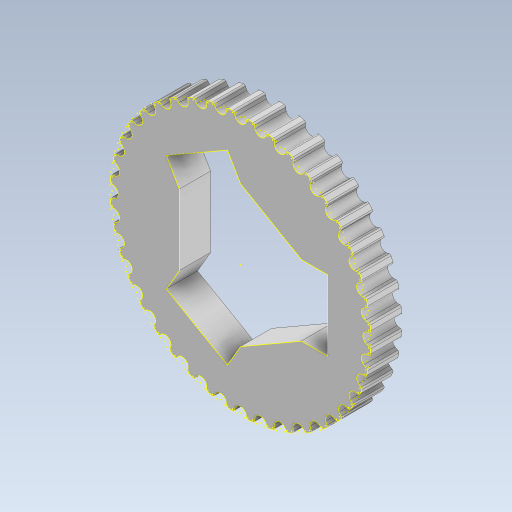
# Autodesk Inventor part: 2GT_40T
Saved by Autodesk Inventor 2023 (Build 270158000, 158)
## iProperties
Created: 2023-05-04
Part Number: 2GT_40T
Material: 一般
Document SubType Name: Modeling
Designer: Johnny Jou
Density: 1 g/cm^3
Appearance: 預設
Author: Johnny Jou
Autodesk Inventor part; units mm, degrees
ref_plane "YZ Plane" through (0, 0, 0) normal (1, 0, 0) x (0, 1, 0)
ref_plane "XZ Plane" through (0, 0, 0) normal (0, 1, 0) x (-1, 0, 0)
ref_plane "XY Plane" through (0, 0, 0) normal (0, 0, 1) x (1, 0, 0)
sketch "草圖1" plane through (0, 0, 0) normal (0, 0, 1) x (1, 0, 0)
  arc A0 (1.3466, 12.2657) -> (1.2112, 12.4161) centre (1.1966, 12.2668) ccw
  arc A1 (1.2112, 12.4161) -> (0.746, 12.4527) centre (0, 0) ccw
  arc A2 (0.746, 12.4527) -> (0.5887, 12.3254) centre (0.7371, 12.3029) ccw
  arc A3 (0.4989, 12.0368) -> (0.5887, 12.3254) centre (-0.4, 12.475) ccw
  arc A4 (-0.4989, 12.0368) -> (0.4989, 12.0368) centre (0, 12.28) ccw
  arc A5 (-0.5887, 12.3254) -> (-0.4989, 12.0368) centre (0.4, 12.475) ccw
  arc A6 (-0.5887, 12.3254) -> (-0.746, 12.4527) centre (-0.7371, 12.3029) ccw
  arc A7 (-0.746, 12.4527) -> (-1.2112, 12.4161) centre (0, 0) ccw
  arc A8 (-1.2112, 12.4161) -> (-1.3466, 12.2657) centre (-1.1966, 12.2668) ccw
  arc A9 (-1.3902, 11.9666) -> (-1.3466, 12.2657) centre (-2.3466, 12.2588) ccw
  arc A10 (-2.3757, 11.8106) -> (-1.3902, 11.9666) centre (-1.921, 12.1288) ccw
  arc A11 (-2.5096, 12.0815) -> (-2.3757, 11.8106) centre (-1.5564, 12.384) ccw
  arc A12 (-2.5096, 12.0815) -> (-2.6849, 12.1827) centre (-2.6526, 12.0362) ccw
  arc A13 (-2.6849, 12.1827) -> (-3.1386, 12.0737) centre (0, 0) ccw
  arc A14 (-3.1386, 12.0737) -> (-3.2488, 11.9041) centre (-3.1008, 11.9286) ccw
  arc A15 (-3.2451, 11.6018) -> (-3.2488, 11.9041) centre (-4.2354, 11.7408) ccw
  arc A16 (-4.194, 11.2935) -> (-3.2451, 11.6018) centre (-3.7947, 11.679) ccw
  arc A17 (-4.3687, 11.5402) -> (-4.194, 11.2935) centre (-3.4746, 11.988) ccw
  arc A18 (-4.3687, 11.5402) -> (-4.5576, 11.6127) centre (-4.5028, 11.473) ccw
  arc A19 (-4.5576, 11.6127) -> (-4.9887, 11.4341) centre (0, 0) ccw
  arc A20 (-4.9887, 11.4341) -> (-5.071, 11.2493) centre (-4.9287, 11.2966) ccw
  arc A21 (-5.0201, 10.9514) -> (-5.071, 11.2493) centre (-6.0199, 10.9337) ccw
  arc A22 (-5.9091, 10.4984) -> (-5.0201, 10.9514) centre (-5.575, 10.9416) ccw
  arc A23 (-6.1202, 10.7147) -> (-5.9091, 10.4984) centre (-5.3071, 11.2969) ccw
  arc A24 (-6.1202, 10.7147) -> (-6.3181, 10.7567) centre (-6.2421, 10.6274) ccw
  arc A25 (-6.3181, 10.7567) -> (-6.7159, 10.5129) centre (0, 0) ccw
  arc A26 (-6.7159, 10.5129) -> (-6.7684, 10.3175) centre (-6.6352, 10.3865) ccw
  arc A27 (-6.6715, 10.0312) -> (-6.7684, 10.3175) centre (-7.6562, 9.8574) ccw
  arc A28 (-7.4787, 9.4447) -> (-6.6715, 10.0312) centre (-7.218, 9.9347) ccw
  arc A29 (-7.721, 9.6254) -> (-7.4787, 9.4447) centre (-7.009, 10.3276) ccw
  arc A30 (-7.721, 9.6254) -> (-7.923, 9.6359) centre (-7.8278, 9.5201) ccw
  arc A31 (-7.923, 9.6359) -> (-8.2778, 9.3329) centre (0, 0) ccw
  arc A32 (-8.2778, 9.3329) -> (-8.2991, 9.1317) centre (-8.1783, 9.2207) ccw
  arc A33 (-8.1585, 8.8641) -> (-8.2991, 9.1317) centre (-9.104, 8.5383) ccw
  arc A34 (-8.8641, 8.1585) -> (-8.1585, 8.8641) centre (-8.6833, 8.6833) ccw
  arc A35 (-9.1317, 8.2991) -> (-8.8641, 8.1585) centre (-8.5383, 9.104) ccw
  arc A36 (-9.1317, 8.2991) -> (-9.3329, 8.2778) centre (-9.2207, 8.1783) ccw
  arc A37 (-9.3329, 8.2778) -> (-9.6359, 7.923) centre (0, 0) ccw
  arc A38 (-9.6359, 7.923) -> (-9.6254, 7.721) centre (-9.5201, 7.8278) ccw
  arc A39 (-9.4447, 7.4787) -> (-9.6254, 7.721) centre (-10.3276, 7.009) ccw
  arc A40 (-10.0312, 6.6715) -> (-9.4447, 7.4787) centre (-9.9347, 7.218) ccw
  arc A41 (-10.3175, 6.7684) -> (-10.0312, 6.6715) centre (-9.8574, 7.6562) ccw
  arc A42 (-10.3175, 6.7684) -> (-10.5129, 6.7159) centre (-10.3865, 6.6352) ccw
  arc A43 (-10.5129, 6.7159) -> (-10.7567, 6.3181) centre (0, 0) ccw
  arc A44 (-10.7567, 6.3181) -> (-10.7147, 6.1202) centre (-10.6274, 6.2421) ccw
  arc A45 (-10.4984, 5.9091) -> (-10.7147, 6.1202) centre (-11.2969, 5.3071) ccw
  arc A46 (-10.9514, 5.0201) -> (-10.4984, 5.9091) centre (-10.9416, 5.575) ccw
  arc A47 (-11.2493, 5.071) -> (-10.9514, 5.0201) centre (-10.9337, 6.0199) ccw
  arc A48 (-11.2493, 5.071) -> (-11.4341, 4.9887) centre (-11.2966, 4.9287) ccw
  arc A49 (-11.4341, 4.9887) -> (-11.6127, 4.5576) centre (0, 0) ccw
  arc A50 (-11.6127, 4.5576) -> (-11.5402, 4.3687) centre (-11.473, 4.5028) ccw
  arc A51 (-11.2935, 4.194) -> (-11.5402, 4.3687) centre (-11.988, 3.4746) ccw
  arc A52 (-11.6018, 3.2451) -> (-11.2935, 4.194) centre (-11.679, 3.7947) ccw
  arc A53 (-11.9041, 3.2488) -> (-11.6018, 3.2451) centre (-11.7408, 4.2354) ccw
  arc A54 (-11.9041, 3.2488) -> (-12.0737, 3.1386) centre (-11.9286, 3.1008) ccw
  arc A55 (-12.0737, 3.1386) -> (-12.1827, 2.6849) centre (0, 0) ccw
  arc A56 (-12.1827, 2.6849) -> (-12.0815, 2.5096) centre (-12.0362, 2.6526) ccw
  arc A57 (-11.8106, 2.3757) -> (-12.0815, 2.5096) centre (-12.384, 1.5564) ccw
  arc A58 (-11.9666, 1.3902) -> (-11.8106, 2.3757) centre (-12.1288, 1.921) ccw
  arc A59 (-12.2657, 1.3466) -> (-11.9666, 1.3902) centre (-12.2588, 2.3466) ccw
  arc A60 (-12.2657, 1.3466) -> (-12.4161, 1.2112) centre (-12.2668, 1.1966) ccw
  arc A61 (-12.4161, 1.2112) -> (-12.4527, 0.746) centre (0, 0) ccw
  arc A62 (-12.4527, 0.746) -> (-12.3254, 0.5887) centre (-12.3029, 0.7371) ccw
  arc A63 (-12.0368, 0.4989) -> (-12.3254, 0.5887) centre (-12.475, -0.4) ccw
  arc A64 (-12.0368, -0.4989) -> (-12.0368, 0.4989) centre (-12.28, 0) ccw
  arc A65 (-12.3254, -0.5887) -> (-12.0368, -0.4989) centre (-12.475, 0.4) ccw
  arc A66 (-12.3254, -0.5887) -> (-12.4527, -0.746) centre (-12.3029, -0.7371) ccw
  arc A67 (-12.4527, -0.746) -> (-12.4161, -1.2112) centre (0, 0) ccw
  arc A68 (-12.4161, -1.2112) -> (-12.2657, -1.3466) centre (-12.2668, -1.1966) ccw
  arc A69 (-11.9666, -1.3902) -> (-12.2657, -1.3466) centre (-12.2588, -2.3466) ccw
  arc A70 (-11.8106, -2.3757) -> (-11.9666, -1.3902) centre (-12.1288, -1.921) ccw
  arc A71 (-12.0815, -2.5096) -> (-11.8106, -2.3757) centre (-12.384, -1.5564) ccw
  arc A72 (-12.0815, -2.5096) -> (-12.1827, -2.6849) centre (-12.0362, -2.6526) ccw
  arc A73 (-12.1827, -2.6849) -> (-12.0737, -3.1386) centre (0, 0) ccw
  arc A74 (-12.0737, -3.1386) -> (-11.9041, -3.2488) centre (-11.9286, -3.1008) ccw
  arc A75 (-11.6018, -3.2451) -> (-11.9041, -3.2488) centre (-11.7408, -4.2354) ccw
  arc A76 (-11.2935, -4.194) -> (-11.6018, -3.2451) centre (-11.679, -3.7947) ccw
  arc A77 (-11.5402, -4.3687) -> (-11.2935, -4.194) centre (-11.988, -3.4746) ccw
  arc A78 (-11.5402, -4.3687) -> (-11.6127, -4.5576) centre (-11.473, -4.5028) ccw
  arc A79 (-11.6127, -4.5576) -> (-11.4341, -4.9887) centre (0, 0) ccw
  arc A80 (-11.4341, -4.9887) -> (-11.2493, -5.071) centre (-11.2966, -4.9287) ccw
  arc A81 (-10.9514, -5.0201) -> (-11.2493, -5.071) centre (-10.9337, -6.0199) ccw
  arc A82 (-10.4984, -5.9091) -> (-10.9514, -5.0201) centre (-10.9416, -5.575) ccw
  arc A83 (-10.7147, -6.1202) -> (-10.4984, -5.9091) centre (-11.2969, -5.3071) ccw
  arc A84 (-10.7147, -6.1202) -> (-10.7567, -6.3181) centre (-10.6274, -6.2421) ccw
  arc A85 (-10.7567, -6.3181) -> (-10.5129, -6.7159) centre (0, 0) ccw
  arc A86 (-10.5129, -6.7159) -> (-10.3175, -6.7684) centre (-10.3865, -6.6352) ccw
  arc A87 (-10.0312, -6.6715) -> (-10.3175, -6.7684) centre (-9.8574, -7.6562) ccw
  arc A88 (-9.4447, -7.4787) -> (-10.0312, -6.6715) centre (-9.9347, -7.218) ccw
  arc A89 (-9.6254, -7.721) -> (-9.4447, -7.4787) centre (-10.3276, -7.009) ccw
  arc A90 (-9.6254, -7.721) -> (-9.6359, -7.923) centre (-9.5201, -7.8278) ccw
  arc A91 (-9.6359, -7.923) -> (-9.3329, -8.2778) centre (0, 0) ccw
  arc A92 (-9.3329, -8.2778) -> (-9.1317, -8.2991) centre (-9.2207, -8.1783) ccw
  arc A93 (-8.8641, -8.1585) -> (-9.1317, -8.2991) centre (-8.5383, -9.104) ccw
  arc A94 (-8.1585, -8.8641) -> (-8.8641, -8.1585) centre (-8.6833, -8.6833) ccw
  arc A95 (-8.2991, -9.1317) -> (-8.1585, -8.8641) centre (-9.104, -8.5383) ccw
  arc A96 (-8.2991, -9.1317) -> (-8.2778, -9.3329) centre (-8.1783, -9.2207) ccw
  arc A97 (-8.2778, -9.3329) -> (-7.923, -9.6359) centre (0, 0) ccw
  arc A98 (-7.923, -9.6359) -> (-7.721, -9.6254) centre (-7.8278, -9.5201) ccw
  arc A99 (-7.4787, -9.4447) -> (-7.721, -9.6254) centre (-7.009, -10.3276) ccw
  arc A100 (-6.6715, -10.0312) -> (-7.4787, -9.4447) centre (-7.218, -9.9347) ccw
  arc A101 (-6.7684, -10.3175) -> (-6.6715, -10.0312) centre (-7.6562, -9.8574) ccw
  arc A102 (-6.7684, -10.3175) -> (-6.7159, -10.5129) centre (-6.6352, -10.3865) ccw
  arc A103 (-6.7159, -10.5129) -> (-6.3181, -10.7567) centre (0, 0) ccw
  arc A104 (-6.3181, -10.7567) -> (-6.1202, -10.7147) centre (-6.2421, -10.6274) ccw
  arc A105 (-5.9091, -10.4984) -> (-6.1202, -10.7147) centre (-5.3071, -11.2969) ccw
  arc A106 (-5.0201, -10.9514) -> (-5.9091, -10.4984) centre (-5.575, -10.9416) ccw
  arc A107 (-5.071, -11.2493) -> (-5.0201, -10.9514) centre (-6.0199, -10.9337) ccw
  arc A108 (-5.071, -11.2493) -> (-4.9887, -11.4341) centre (-4.9287, -11.2966) ccw
  arc A109 (-4.9887, -11.4341) -> (-4.5576, -11.6127) centre (0, 0) ccw
  arc A110 (-4.5576, -11.6127) -> (-4.3687, -11.5402) centre (-4.5028, -11.473) ccw
  arc A111 (-4.194, -11.2935) -> (-4.3687, -11.5402) centre (-3.4746, -11.988) ccw
  arc A112 (-3.2451, -11.6018) -> (-4.194, -11.2935) centre (-3.7947, -11.679) ccw
  arc A113 (-3.2488, -11.9041) -> (-3.2451, -11.6018) centre (-4.2354, -11.7408) ccw
  arc A114 (-3.2488, -11.9041) -> (-3.1386, -12.0737) centre (-3.1008, -11.9286) ccw
  arc A115 (-3.1386, -12.0737) -> (-2.6849, -12.1827) centre (0, 0) ccw
  arc A116 (-2.6849, -12.1827) -> (-2.5096, -12.0815) centre (-2.6526, -12.0362) ccw
  arc A117 (-2.3757, -11.8106) -> (-2.5096, -12.0815) centre (-1.5564, -12.384) ccw
  arc A118 (-1.3902, -11.9666) -> (-2.3757, -11.8106) centre (-1.921, -12.1288) ccw
  arc A119 (-1.3466, -12.2657) -> (-1.3902, -11.9666) centre (-2.3466, -12.2588) ccw
  arc A120 (-1.3466, -12.2657) -> (-1.2112, -12.4161) centre (-1.1966, -12.2668) ccw
  arc A121 (-1.2112, -12.4161) -> (-0.746, -12.4527) centre (0, 0) ccw
  arc A122 (-0.746, -12.4527) -> (-0.5887, -12.3254) centre (-0.7371, -12.3029) ccw
  arc A123 (-0.4989, -12.0368) -> (-0.5887, -12.3254) centre (0.4, -12.475) ccw
  arc A124 (0.4989, -12.0368) -> (-0.4989, -12.0368) centre (0, -12.28) ccw
  arc A125 (0.5887, -12.3254) -> (0.4989, -12.0368) centre (-0.4, -12.475) ccw
  arc A126 (0.5887, -12.3254) -> (0.746, -12.4527) centre (0.7371, -12.3029) ccw
  arc A127 (0.746, -12.4527) -> (1.2112, -12.4161) centre (0, 0) ccw
  arc A128 (1.2112, -12.4161) -> (1.3466, -12.2657) centre (1.1966, -12.2668) ccw
  arc A129 (1.3902, -11.9666) -> (1.3466, -12.2657) centre (2.3466, -12.2588) ccw
  arc A130 (2.3757, -11.8106) -> (1.3902, -11.9666) centre (1.921, -12.1288) ccw
  arc A131 (2.5096, -12.0815) -> (2.3757, -11.8106) centre (1.5564, -12.384) ccw
  arc A132 (2.5096, -12.0815) -> (2.6849, -12.1827) centre (2.6526, -12.0362) ccw
  arc A133 (2.6849, -12.1827) -> (3.1386, -12.0737) centre (0, 0) ccw
  arc A134 (3.1386, -12.0737) -> (3.2488, -11.9041) centre (3.1008, -11.9286) ccw
  arc A135 (3.2451, -11.6018) -> (3.2488, -11.9041) centre (4.2354, -11.7408) ccw
  arc A136 (4.194, -11.2935) -> (3.2451, -11.6018) centre (3.7947, -11.679) ccw
  arc A137 (4.3687, -11.5402) -> (4.194, -11.2935) centre (3.4746, -11.988) ccw
  arc A138 (4.3687, -11.5402) -> (4.5576, -11.6127) centre (4.5028, -11.473) ccw
  arc A139 (4.5576, -11.6127) -> (4.9887, -11.4341) centre (0, 0) ccw
  arc A140 (4.9887, -11.4341) -> (5.071, -11.2493) centre (4.9287, -11.2966) ccw
  arc A141 (5.0201, -10.9514) -> (5.071, -11.2493) centre (6.0199, -10.9337) ccw
  arc A142 (5.9091, -10.4984) -> (5.0201, -10.9514) centre (5.575, -10.9416) ccw
  arc A143 (6.1202, -10.7147) -> (5.9091, -10.4984) centre (5.3071, -11.2969) ccw
  arc A144 (6.1202, -10.7147) -> (6.3181, -10.7567) centre (6.2421, -10.6274) ccw
  arc A145 (6.3181, -10.7567) -> (6.7159, -10.5129) centre (0, 0) ccw
  arc A146 (6.7159, -10.5129) -> (6.7684, -10.3175) centre (6.6352, -10.3865) ccw
  arc A147 (6.6715, -10.0312) -> (6.7684, -10.3175) centre (7.6562, -9.8574) ccw
  arc A148 (7.4787, -9.4447) -> (6.6715, -10.0312) centre (7.218, -9.9347) ccw
  arc A149 (7.721, -9.6254) -> (7.4787, -9.4447) centre (7.009, -10.3276) ccw
  arc A150 (7.721, -9.6254) -> (7.923, -9.6359) centre (7.8278, -9.5201) ccw
  arc A151 (7.923, -9.6359) -> (8.2778, -9.3329) centre (0, 0) ccw
  arc A152 (8.2778, -9.3329) -> (8.2991, -9.1317) centre (8.1783, -9.2207) ccw
  arc A153 (8.1585, -8.8641) -> (8.2991, -9.1317) centre (9.104, -8.5383) ccw
  arc A154 (8.8641, -8.1585) -> (8.1585, -8.8641) centre (8.6833, -8.6833) ccw
  arc A155 (9.1317, -8.2991) -> (8.8641, -8.1585) centre (8.5383, -9.104) ccw
  arc A156 (9.1317, -8.2991) -> (9.3329, -8.2778) centre (9.2207, -8.1783) ccw
  arc A157 (9.3329, -8.2778) -> (9.6359, -7.923) centre (0, 0) ccw
  arc A158 (9.6359, -7.923) -> (9.6254, -7.721) centre (9.5201, -7.8278) ccw
  arc A159 (9.4447, -7.4787) -> (9.6254, -7.721) centre (10.3276, -7.009) ccw
  arc A160 (10.0312, -6.6715) -> (9.4447, -7.4787) centre (9.9347, -7.218) ccw
  arc A161 (10.3175, -6.7684) -> (10.0312, -6.6715) centre (9.8574, -7.6562) ccw
  arc A162 (10.3175, -6.7684) -> (10.5129, -6.7159) centre (10.3865, -6.6352) ccw
  arc A163 (10.5129, -6.7159) -> (10.7567, -6.3181) centre (0, 0) ccw
  arc A164 (10.7567, -6.3181) -> (10.7147, -6.1202) centre (10.6274, -6.2421) ccw
  arc A165 (10.4984, -5.9091) -> (10.7147, -6.1202) centre (11.2969, -5.3071) ccw
  arc A166 (10.9514, -5.0201) -> (10.4984, -5.9091) centre (10.9416, -5.575) ccw
  arc A167 (11.2493, -5.071) -> (10.9514, -5.0201) centre (10.9337, -6.0199) ccw
  arc A168 (11.2493, -5.071) -> (11.4341, -4.9887) centre (11.2966, -4.9287) ccw
  arc A169 (11.4341, -4.9887) -> (11.6127, -4.5576) centre (0, 0) ccw
  arc A170 (11.6127, -4.5576) -> (11.5402, -4.3687) centre (11.473, -4.5028) ccw
  arc A171 (11.2935, -4.194) -> (11.5402, -4.3687) centre (11.988, -3.4746) ccw
  arc A172 (11.6018, -3.2451) -> (11.2935, -4.194) centre (11.679, -3.7947) ccw
  arc A173 (11.9041, -3.2488) -> (11.6018, -3.2451) centre (11.7408, -4.2354) ccw
  arc A174 (11.9041, -3.2488) -> (12.0737, -3.1386) centre (11.9286, -3.1008) ccw
  arc A175 (12.0737, -3.1386) -> (12.1827, -2.6849) centre (0, 0) ccw
  arc A176 (12.1827, -2.6849) -> (12.0815, -2.5096) centre (12.0362, -2.6526) ccw
  arc A177 (11.8106, -2.3757) -> (12.0815, -2.5096) centre (12.384, -1.5564) ccw
  arc A178 (11.9666, -1.3902) -> (11.8106, -2.3757) centre (12.1288, -1.921) ccw
  arc A179 (12.2657, -1.3466) -> (11.9666, -1.3902) centre (12.2588, -2.3466) ccw
  arc A180 (12.2657, -1.3466) -> (12.4161, -1.2112) centre (12.2668, -1.1966) ccw
  arc A181 (12.4161, -1.2112) -> (12.4527, -0.746) centre (0, 0) ccw
  arc A182 (12.4527, -0.746) -> (12.3254, -0.5887) centre (12.3029, -0.7371) ccw
  arc A183 (12.0368, -0.4989) -> (12.3254, -0.5887) centre (12.475, 0.4) ccw
  arc A184 (12.0368, 0.4989) -> (12.0368, -0.4989) centre (12.28, 0) ccw
  arc A185 (12.3254, 0.5887) -> (12.0368, 0.4989) centre (12.475, -0.4) ccw
  arc A186 (12.3254, 0.5887) -> (12.4527, 0.746) centre (12.3029, 0.7371) ccw
  arc A187 (12.4527, 0.746) -> (12.4161, 1.2112) centre (0, 0) ccw
  arc A188 (12.4161, 1.2112) -> (12.2657, 1.3466) centre (12.2668, 1.1966) ccw
  arc A189 (11.9666, 1.3902) -> (12.2657, 1.3466) centre (12.2588, 2.3466) ccw
  arc A190 (11.8106, 2.3757) -> (11.9666, 1.3902) centre (12.1288, 1.921) ccw
  arc A191 (12.0815, 2.5096) -> (11.8106, 2.3757) centre (12.384, 1.5564) ccw
  arc A192 (12.0815, 2.5096) -> (12.1827, 2.6849) centre (12.0362, 2.6526) ccw
  arc A193 (12.1827, 2.6849) -> (12.0737, 3.1386) centre (0, 0) ccw
  arc A194 (12.0737, 3.1386) -> (11.9041, 3.2488) centre (11.9286, 3.1008) ccw
  arc A195 (11.6018, 3.2451) -> (11.9041, 3.2488) centre (11.7408, 4.2354) ccw
  arc A196 (11.2935, 4.194) -> (11.6018, 3.2451) centre (11.679, 3.7947) ccw
  arc A197 (11.5402, 4.3687) -> (11.2935, 4.194) centre (11.988, 3.4746) ccw
  arc A198 (11.5402, 4.3687) -> (11.6127, 4.5576) centre (11.473, 4.5028) ccw
  arc A199 (11.6127, 4.5576) -> (11.4341, 4.9887) centre (0, 0) ccw
  arc A200 (11.4341, 4.9887) -> (11.2493, 5.071) centre (11.2966, 4.9287) ccw
  arc A201 (10.9514, 5.0201) -> (11.2493, 5.071) centre (10.9337, 6.0199) ccw
  arc A202 (10.4984, 5.9091) -> (10.9514, 5.0201) centre (10.9416, 5.575) ccw
  arc A203 (10.7147, 6.1202) -> (10.4984, 5.9091) centre (11.2969, 5.3071) ccw
  arc A204 (10.7147, 6.1202) -> (10.7567, 6.3181) centre (10.6274, 6.2421) ccw
  arc A205 (10.7567, 6.3181) -> (10.5129, 6.7159) centre (0, 0) ccw
  arc A206 (10.5129, 6.7159) -> (10.3175, 6.7684) centre (10.3865, 6.6352) ccw
  arc A207 (10.0312, 6.6715) -> (10.3175, 6.7684) centre (9.8574, 7.6562) ccw
  arc A208 (9.4447, 7.4787) -> (10.0312, 6.6715) centre (9.9347, 7.218) ccw
  arc A209 (9.6254, 7.721) -> (9.4447, 7.4787) centre (10.3276, 7.009) ccw
  arc A210 (9.6254, 7.721) -> (9.6359, 7.923) centre (9.5201, 7.8278) ccw
  arc A211 (9.6359, 7.923) -> (9.3329, 8.2778) centre (0, 0) ccw
  arc A212 (9.3329, 8.2778) -> (9.1317, 8.2991) centre (9.2207, 8.1783) ccw
  arc A213 (8.8641, 8.1585) -> (9.1317, 8.2991) centre (8.5383, 9.104) ccw
  arc A214 (8.1585, 8.8641) -> (8.8641, 8.1585) centre (8.6833, 8.6833) ccw
  arc A215 (8.2991, 9.1317) -> (8.1585, 8.8641) centre (9.104, 8.5383) ccw
  arc A216 (8.2991, 9.1317) -> (8.2778, 9.3329) centre (8.1783, 9.2207) ccw
  arc A217 (8.2778, 9.3329) -> (7.923, 9.6359) centre (0, 0) ccw
  arc A218 (7.923, 9.6359) -> (7.721, 9.6254) centre (7.8278, 9.5201) ccw
  arc A219 (7.4787, 9.4447) -> (7.721, 9.6254) centre (7.009, 10.3276) ccw
  arc A220 (6.6715, 10.0312) -> (7.4787, 9.4447) centre (7.218, 9.9347) ccw
  arc A221 (6.7684, 10.3175) -> (6.6715, 10.0312) centre (7.6562, 9.8574) ccw
  arc A222 (6.7684, 10.3175) -> (6.7159, 10.5129) centre (6.6352, 10.3865) ccw
  arc A223 (6.7159, 10.5129) -> (6.3181, 10.7567) centre (0, 0) ccw
  arc A224 (6.3181, 10.7567) -> (6.1202, 10.7147) centre (6.2421, 10.6274) ccw
  arc A225 (5.9091, 10.4984) -> (6.1202, 10.7147) centre (5.3071, 11.2969) ccw
  arc A226 (5.0201, 10.9514) -> (5.9091, 10.4984) centre (5.575, 10.9416) ccw
  arc A227 (5.071, 11.2493) -> (5.0201, 10.9514) centre (6.0199, 10.9337) ccw
  arc A228 (5.071, 11.2493) -> (4.9887, 11.4341) centre (4.9287, 11.2966) ccw
  arc A229 (4.9887, 11.4341) -> (4.5576, 11.6127) centre (0, 0) ccw
  arc A230 (4.5576, 11.6127) -> (4.3687, 11.5402) centre (4.5028, 11.473) ccw
  arc A231 (4.194, 11.2935) -> (4.3687, 11.5402) centre (3.4746, 11.988) ccw
  arc A232 (3.2451, 11.6018) -> (4.194, 11.2935) centre (3.7947, 11.679) ccw
  arc A233 (3.2488, 11.9041) -> (3.2451, 11.6018) centre (4.2354, 11.7408) ccw
  arc A234 (3.2488, 11.9041) -> (3.1386, 12.0737) centre (3.1008, 11.9286) ccw
  arc A235 (3.1386, 12.0737) -> (2.6849, 12.1827) centre (0, 0) ccw
  arc A236 (2.6849, 12.1827) -> (2.5096, 12.0815) centre (2.6526, 12.0362) ccw
  arc A237 (2.3757, 11.8106) -> (2.5096, 12.0815) centre (1.5564, 12.384) ccw
  arc A238 (1.3902, 11.9666) -> (2.3757, 11.8106) centre (1.921, 12.1288) ccw
  arc A239 (1.3466, 12.2657) -> (1.3902, 11.9666) centre (2.3466, 12.2588) ccw
  line L0 (-2.5, 7.899) -> (2.5, 7.899)
  line L1 (2.5, 7.899) -> (2.5, 4.899)
  line L2 (-2.5, 4.899) -> (-2.5, 7.899)
  line L3 (8.0907, -1.7844) -> (5.5907, -6.1146)
  line L4 (5.4926, -0.2844) -> (8.0907, -1.7844)
  line L5 (5.5907, -6.1146) -> (2.9926, -4.6146)
  line L6 (-5.5907, -6.1146) -> (-8.0907, -1.7844)
  line L7 (-2.9926, -4.6146) -> (-5.5907, -6.1146)
  line L8 (-8.0907, -1.7844) -> (-5.4926, -0.2844)
  dimension "d7" = 360
  constraints: 480 point on circle, 240 centre point, 18 end point, 2 coincident, 1 horizontal, 1 parallel, 1 perpendicular, 703 other
extrude "擠出1" add sketch "草圖1" along normal blind 3
sketch "草圖2" plane through (0, 0, 0) normal (0, 0, -1) x (-1, 0, 0)
  line L0 (-5.85, -3.3775) -> (-5.85, 3.3775)
  line L1 (-5.85, 3.3775) -> (0, 6.755)
  line L2 (0, 6.755) -> (5.85, 3.3775)
  line L3 (5.85, 3.3775) -> (5.85, -3.3775)
  line L4 (5.85, -3.3775) -> (0, -6.755)
  line L5 (0, -6.755) -> (-5.85, -3.3775)
  line L6 (-5.85, 3.3775) -> (-5.85, -3.3775)
  line L7 (-5.85, -3.3775) -> (-8.35, -3.3775)
  line L8 (-8.35, -3.3775) -> (-8.35, 3.3775)
  line L9 (-8.35, 3.3775) -> (-5.85, 3.3775)
  line L10 (7.1, -5.5426) -> (1.25, -8.9201)
  line L11 (1.25, -8.9201) -> (0, -6.755)
  line L12 (5.85, -3.3775) -> (7.1, -5.5426)
  line L13 (1.25, 8.9201) -> (7.1, 5.5426)
  line L14 (7.1, 5.5426) -> (5.85, 3.3775)
  line L15 (0, 6.755) -> (1.25, 8.9201)
  point P0 (0, 0)
  point P1 (0, 0)
  point P2 (-5.85, 0)
  point P3 (0, -6.755)
  point P4 (5.85, -3.3775)
  point P5 (0, 6.755)
  dimension "d9" = 11.7
  dimension "d10" = 2.5
  dimension "d13" = 360
  constraints: 32 end point, 3 equal length, 1 coincident, 1 midpoint, 1 perpendicular, 1 vertical, 35 other
  measures "d9" distance between parallel lines of L0 L3
  measures "d10" distance of L0.start L7.end
extrude "擠出2" cut sketch "草圖2" against normal up to surface (3 mm away)
sketch "草圖3" plane through (0, 0, 3) normal (0, 0, 1) x (1, 0, 0)
  line L0 (0, 6.755) -> (5.85, 3.3775) projected
  line L1 (5.85, 3.3775) -> (8.35, 3.3775) projected
  line L2 (8.35, 3.3775) -> (8.35, -3.3775) projected
  line L3 (8.35, -3.3775) -> (5.85, -3.3775) projected
  line L4 (5.85, -3.3775) -> (0, -6.755) projected
  line L5 (0, -6.755) -> (-1.25, -8.9201) projected
  line L6 (-1.25, -8.9201) -> (-7.1, -5.5426) projected
  line L7 (-7.1, -5.5426) -> (-5.85, -3.3775) projected
  line L8 (-5.85, -3.3775) -> (-5.85, 3.3775) projected
  line L9 (-5.85, 3.3775) -> (-7.1, 5.5426) projected
  line L10 (-7.1, 5.5426) -> (-1.25, 8.9201) projected
  line L11 (-1.25, 8.9201) -> (0, 6.755) projected
  arc A0 (-4.5576, 11.6127) -> (-4.9887, 11.4341) centre (0, 0) ccw projected
  arc A1 (-4.9887, 11.4341) -> (-5.071, 11.2493) centre (-4.9287, 11.2966) ccw projected
  arc A2 (-5.0201, 10.9514) -> (-5.071, 11.2493) centre (-6.0199, 10.9337) ccw projected
  arc A3 (-5.9091, 10.4984) -> (-5.0201, 10.9514) centre (-5.575, 10.9416) ccw projected
  arc A4 (-6.1202, 10.7147) -> (-5.9091, 10.4984) centre (-5.3071, 11.2969) ccw projected
  arc A5 (-6.1202, 10.7147) -> (-6.3181, 10.7567) centre (-6.2421, 10.6274) ccw projected
  arc A6 (-6.3181, 10.7567) -> (-6.7159, 10.5129) centre (0, 0) ccw projected
  arc A7 (-6.7159, 10.5129) -> (-6.7684, 10.3175) centre (-6.6352, 10.3865) ccw projected
  arc A8 (-6.6715, 10.0312) -> (-6.7684, 10.3175) centre (-7.6562, 9.8574) ccw projected
  arc A9 (-7.4787, 9.4447) -> (-6.6715, 10.0312) centre (-7.218, 9.9347) ccw projected
  arc A10 (-7.721, 9.6254) -> (-7.4787, 9.4447) centre (-7.009, 10.3276) ccw projected
  arc A11 (-7.721, 9.6254) -> (-7.923, 9.6359) centre (-7.8278, 9.5201) ccw projected
  arc A12 (-7.923, 9.6359) -> (-8.2778, 9.3329) centre (0, 0) ccw projected
  arc A13 (-8.2778, 9.3329) -> (-8.2991, 9.1317) centre (-8.1783, 9.2207) ccw projected
  arc A14 (-8.1585, 8.8641) -> (-8.2991, 9.1317) centre (-9.104, 8.5383) ccw projected
  arc A15 (-8.8641, 8.1585) -> (-8.1585, 8.8641) centre (-8.6833, 8.6833) ccw projected
  arc A16 (-9.1317, 8.2991) -> (-8.8641, 8.1585) centre (-8.5383, 9.104) ccw projected
  arc A17 (-9.1317, 8.2991) -> (-9.3329, 8.2778) centre (-9.2207, 8.1783) ccw projected
  arc A18 (-9.3329, 8.2778) -> (-9.6359, 7.923) centre (0, 0) ccw projected
  arc A19 (-9.6359, 7.923) -> (-9.6254, 7.721) centre (-9.5201, 7.8278) ccw projected
  arc A20 (-9.4447, 7.4787) -> (-9.6254, 7.721) centre (-10.3276, 7.009) ccw projected
  arc A21 (-10.0312, 6.6715) -> (-9.4447, 7.4787) centre (-9.9347, 7.218) ccw projected
  arc A22 (-10.3175, 6.7684) -> (-10.0312, 6.6715) centre (-9.8574, 7.6562) ccw projected
  arc A23 (-10.3175, 6.7684) -> (-10.5129, 6.7159) centre (-10.3865, 6.6352) ccw projected
  arc A24 (-10.5129, 6.7159) -> (-10.7567, 6.3181) centre (0, 0) ccw projected
  arc A25 (-10.7567, 6.3181) -> (-10.7147, 6.1202) centre (-10.6274, 6.2421) ccw projected
  arc A26 (-10.4984, 5.9091) -> (-10.7147, 6.1202) centre (-11.2969, 5.3071) ccw projected
  arc A27 (-10.9514, 5.0201) -> (-10.4984, 5.9091) centre (-10.9416, 5.575) ccw projected
  arc A28 (-11.2493, 5.071) -> (-10.9514, 5.0201) centre (-10.9337, 6.0199) ccw projected
  arc A29 (-11.2493, 5.071) -> (-11.4341, 4.9887) centre (-11.2966, 4.9287) ccw projected
  arc A30 (-11.4341, 4.9887) -> (-11.6127, 4.5576) centre (0, 0) ccw projected
  arc A31 (-11.6127, 4.5576) -> (-11.5402, 4.3687) centre (-11.473, 4.5028) ccw projected
  arc A32 (-11.2935, 4.194) -> (-11.5402, 4.3687) centre (-11.988, 3.4746) ccw projected
  arc A33 (-11.6018, 3.2451) -> (-11.2935, 4.194) centre (-11.679, 3.7947) ccw projected
  arc A34 (-11.9041, 3.2488) -> (-11.6018, 3.2451) centre (-11.7408, 4.2354) ccw projected
  arc A35 (-11.9041, 3.2488) -> (-12.0737, 3.1386) centre (-11.9286, 3.1008) ccw projected
  arc A36 (-12.0737, 3.1386) -> (-12.1827, 2.6849) centre (0, 0) ccw projected
  arc A37 (-12.1827, 2.6849) -> (-12.0815, 2.5096) centre (-12.0362, 2.6526) ccw projected
  arc A38 (-11.8106, 2.3757) -> (-12.0815, 2.5096) centre (-12.384, 1.5564) ccw projected
  arc A39 (-11.9666, 1.3902) -> (-11.8106, 2.3757) centre (-12.1288, 1.921) ccw projected
  arc A40 (-12.2657, 1.3466) -> (-11.9666, 1.3902) centre (-12.2588, 2.3466) ccw projected
  arc A41 (-12.2657, 1.3466) -> (-12.4161, 1.2112) centre (-12.2668, 1.1966) ccw projected
  arc A42 (-12.4161, 1.2112) -> (-12.4527, 0.746) centre (0, 0) ccw projected
  arc A43 (-12.4527, 0.746) -> (-12.3254, 0.5887) centre (-12.3029, 0.7371) ccw projected
  arc A44 (-12.0368, 0.4989) -> (-12.3254, 0.5887) centre (-12.475, -0.4) ccw projected
  arc A45 (-12.0368, -0.4989) -> (-12.0368, 0.4989) centre (-12.28, 0) ccw projected
  arc A46 (-12.3254, -0.5887) -> (-12.0368, -0.4989) centre (-12.475, 0.4) ccw projected
  arc A47 (-12.3254, -0.5887) -> (-12.4527, -0.746) centre (-12.3029, -0.7371) ccw projected
  arc A48 (-12.4527, -0.746) -> (-12.4161, -1.2112) centre (0, 0) ccw projected
  arc A49 (-12.4161, -1.2112) -> (-12.2657, -1.3466) centre (-12.2668, -1.1966) ccw projected
  arc A50 (-11.9666, -1.3902) -> (-12.2657, -1.3466) centre (-12.2588, -2.3466) ccw projected
  arc A51 (-11.8106, -2.3757) -> (-11.9666, -1.3902) centre (-12.1288, -1.921) ccw projected
  arc A52 (-12.0815, -2.5096) -> (-11.8106, -2.3757) centre (-12.384, -1.5564) ccw projected
  arc A53 (-12.0815, -2.5096) -> (-12.1827, -2.6849) centre (-12.0362, -2.6526) ccw projected
  arc A54 (-12.1827, -2.6849) -> (-12.0737, -3.1386) centre (0, 0) ccw projected
  arc A55 (-12.0737, -3.1386) -> (-11.9041, -3.2488) centre (-11.9286, -3.1008) ccw projected
  arc A56 (-11.6018, -3.2451) -> (-11.9041, -3.2488) centre (-11.7408, -4.2354) ccw projected
  arc A57 (-11.2935, -4.194) -> (-11.6018, -3.2451) centre (-11.679, -3.7947) ccw projected
  arc A58 (-11.5402, -4.3687) -> (-11.2935, -4.194) centre (-11.988, -3.4746) ccw projected
  arc A59 (-11.5402, -4.3687) -> (-11.6127, -4.5576) centre (-11.473, -4.5028) ccw projected
  arc A60 (-11.6127, -4.5576) -> (-11.4341, -4.9887) centre (0, 0) ccw projected
  arc A61 (-11.4341, -4.9887) -> (-11.2493, -5.071) centre (-11.2966, -4.9287) ccw projected
  arc A62 (-10.9514, -5.0201) -> (-11.2493, -5.071) centre (-10.9337, -6.0199) ccw projected
  arc A63 (-10.4984, -5.9091) -> (-10.9514, -5.0201) centre (-10.9416, -5.575) ccw projected
  arc A64 (-10.7147, -6.1202) -> (-10.4984, -5.9091) centre (-11.2969, -5.3071) ccw projected
  arc A65 (-10.7147, -6.1202) -> (-10.7567, -6.3181) centre (-10.6274, -6.2421) ccw projected
  arc A66 (-10.7567, -6.3181) -> (-10.5129, -6.7159) centre (0, 0) ccw projected
  arc A67 (-10.5129, -6.7159) -> (-10.3175, -6.7684) centre (-10.3865, -6.6352) ccw projected
  arc A68 (-10.0312, -6.6715) -> (-10.3175, -6.7684) centre (-9.8574, -7.6562) ccw projected
  arc A69 (-9.4447, -7.4787) -> (-10.0312, -6.6715) centre (-9.9347, -7.218) ccw projected
  arc A70 (-9.6254, -7.721) -> (-9.4447, -7.4787) centre (-10.3276, -7.009) ccw projected
  arc A71 (-9.6254, -7.721) -> (-9.6359, -7.923) centre (-9.5201, -7.8278) ccw projected
  arc A72 (-9.6359, -7.923) -> (-9.3329, -8.2778) centre (0, 0) ccw projected
  arc A73 (-9.3329, -8.2778) -> (-9.1317, -8.2991) centre (-9.2207, -8.1783) ccw projected
  arc A74 (-8.8641, -8.1585) -> (-9.1317, -8.2991) centre (-8.5383, -9.104) ccw projected
  arc A75 (-8.1585, -8.8641) -> (-8.8641, -8.1585) centre (-8.6833, -8.6833) ccw projected
  arc A76 (-8.2991, -9.1317) -> (-8.1585, -8.8641) centre (-9.104, -8.5383) ccw projected
  arc A77 (-8.2991, -9.1317) -> (-8.2778, -9.3329) centre (-8.1783, -9.2207) ccw projected
  arc A78 (-8.2778, -9.3329) -> (-7.923, -9.6359) centre (0, 0) ccw projected
  arc A79 (-7.923, -9.6359) -> (-7.721, -9.6254) centre (-7.8278, -9.5201) ccw projected
  arc A80 (-7.4787, -9.4447) -> (-7.721, -9.6254) centre (-7.009, -10.3276) ccw projected
  arc A81 (-6.6715, -10.0312) -> (-7.4787, -9.4447) centre (-7.218, -9.9347) ccw projected
  arc A82 (-6.7684, -10.3175) -> (-6.6715, -10.0312) centre (-7.6562, -9.8574) ccw projected
  arc A83 (-6.7684, -10.3175) -> (-6.7159, -10.5129) centre (-6.6352, -10.3865) ccw projected
  arc A84 (-6.7159, -10.5129) -> (-6.3181, -10.7567) centre (0, 0) ccw projected
  arc A85 (-6.3181, -10.7567) -> (-6.1202, -10.7147) centre (-6.2421, -10.6274) ccw projected
  arc A86 (-5.9091, -10.4984) -> (-6.1202, -10.7147) centre (-5.3071, -11.2969) ccw projected
  arc A87 (-5.0201, -10.9514) -> (-5.9091, -10.4984) centre (-5.575, -10.9416) ccw projected
  arc A88 (-5.071, -11.2493) -> (-5.0201, -10.9514) centre (-6.0199, -10.9337) ccw projected
  arc A89 (-5.071, -11.2493) -> (-4.9887, -11.4341) centre (-4.9287, -11.2966) ccw projected
  arc A90 (-4.9887, -11.4341) -> (-4.5576, -11.6127) centre (0, 0) ccw projected
  arc A91 (-4.5576, -11.6127) -> (-4.3687, -11.5402) centre (-4.5028, -11.473) ccw projected
  arc A92 (-4.194, -11.2935) -> (-4.3687, -11.5402) centre (-3.4746, -11.988) ccw projected
  arc A93 (-3.2451, -11.6018) -> (-4.194, -11.2935) centre (-3.7947, -11.679) ccw projected
  arc A94 (-3.2488, -11.9041) -> (-3.2451, -11.6018) centre (-4.2354, -11.7408) ccw projected
  arc A95 (-3.2488, -11.9041) -> (-3.1386, -12.0737) centre (-3.1008, -11.9286) ccw projected
  arc A96 (-3.1386, -12.0737) -> (-2.6849, -12.1827) centre (0, 0) ccw projected
  arc A97 (-2.6849, -12.1827) -> (-2.5096, -12.0815) centre (-2.6526, -12.0362) ccw projected
  arc A98 (-2.3757, -11.8106) -> (-2.5096, -12.0815) centre (-1.5564, -12.384) ccw projected
  arc A99 (-1.3902, -11.9666) -> (-2.3757, -11.8106) centre (-1.921, -12.1288) ccw projected
  arc A100 (-1.3466, -12.2657) -> (-1.3902, -11.9666) centre (-2.3466, -12.2588) ccw projected
  arc A101 (-1.3466, -12.2657) -> (-1.2112, -12.4161) centre (-1.1966, -12.2668) ccw projected
  arc A102 (-1.2112, -12.4161) -> (-0.746, -12.4527) centre (0, 0) ccw projected
  arc A103 (-0.746, -12.4527) -> (-0.5887, -12.3254) centre (-0.7371, -12.3029) ccw projected
  arc A104 (-0.4989, -12.0368) -> (-0.5887, -12.3254) centre (0.4, -12.475) ccw projected
  arc A105 (0.4989, -12.0368) -> (-0.4989, -12.0368) centre (0, -12.28) ccw projected
  arc A106 (0.5887, -12.3254) -> (0.4989, -12.0368) centre (-0.4, -12.475) ccw projected
  arc A107 (0.5887, -12.3254) -> (0.746, -12.4527) centre (0.7371, -12.3029) ccw projected
  arc A108 (0.746, -12.4527) -> (1.2112, -12.4161) centre (0, 0) ccw projected
  arc A109 (1.2112, -12.4161) -> (1.3466, -12.2657) centre (1.1966, -12.2668) ccw projected
  arc A110 (1.3902, -11.9666) -> (1.3466, -12.2657) centre (2.3466, -12.2588) ccw projected
  arc A111 (2.3757, -11.8106) -> (1.3902, -11.9666) centre (1.921, -12.1288) ccw projected
  arc A112 (2.5096, -12.0815) -> (2.3757, -11.8106) centre (1.5564, -12.384) ccw projected
  arc A113 (2.5096, -12.0815) -> (2.6849, -12.1827) centre (2.6526, -12.0362) ccw projected
  arc A114 (2.6849, -12.1827) -> (3.1386, -12.0737) centre (0, 0) ccw projected
  arc A115 (3.1386, -12.0737) -> (3.2488, -11.9041) centre (3.1008, -11.9286) ccw projected
  arc A116 (3.2451, -11.6018) -> (3.2488, -11.9041) centre (4.2354, -11.7408) ccw projected
  arc A117 (4.194, -11.2935) -> (3.2451, -11.6018) centre (3.7947, -11.679) ccw projected
  arc A118 (4.3687, -11.5402) -> (4.194, -11.2935) centre (3.4746, -11.988) ccw projected
  arc A119 (4.3687, -11.5402) -> (4.5576, -11.6127) centre (4.5028, -11.473) ccw projected
  arc A120 (4.5576, -11.6127) -> (4.9887, -11.4341) centre (0, 0) ccw projected
  arc A121 (4.9887, -11.4341) -> (5.071, -11.2493) centre (4.9287, -11.2966) ccw projected
  arc A122 (5.0201, -10.9514) -> (5.071, -11.2493) centre (6.0199, -10.9337) ccw projected
  arc A123 (5.9091, -10.4984) -> (5.0201, -10.9514) centre (5.575, -10.9416) ccw projected
  arc A124 (6.1202, -10.7147) -> (5.9091, -10.4984) centre (5.3071, -11.2969) ccw projected
  arc A125 (6.1202, -10.7147) -> (6.3181, -10.7567) centre (6.2421, -10.6274) ccw projected
  arc A126 (6.3181, -10.7567) -> (6.7159, -10.5129) centre (0, 0) ccw projected
  arc A127 (6.7159, -10.5129) -> (6.7684, -10.3175) centre (6.6352, -10.3865) ccw projected
  arc A128 (6.6715, -10.0312) -> (6.7684, -10.3175) centre (7.6562, -9.8574) ccw projected
  arc A129 (7.4787, -9.4447) -> (6.6715, -10.0312) centre (7.218, -9.9347) ccw projected
  arc A130 (7.721, -9.6254) -> (7.4787, -9.4447) centre (7.009, -10.3276) ccw projected
  arc A131 (7.721, -9.6254) -> (7.923, -9.6359) centre (7.8278, -9.5201) ccw projected
  arc A132 (7.923, -9.6359) -> (8.2778, -9.3329) centre (0, 0) ccw projected
  arc A133 (8.2778, -9.3329) -> (8.2991, -9.1317) centre (8.1783, -9.2207) ccw projected
  arc A134 (8.1585, -8.8641) -> (8.2991, -9.1317) centre (9.104, -8.5383) ccw projected
  arc A135 (8.8641, -8.1585) -> (8.1585, -8.8641) centre (8.6833, -8.6833) ccw projected
  arc A136 (9.1317, -8.2991) -> (8.8641, -8.1585) centre (8.5383, -9.104) ccw projected
  arc A137 (9.1317, -8.2991) -> (9.3329, -8.2778) centre (9.2207, -8.1783) ccw projected
  arc A138 (9.3329, -8.2778) -> (9.6359, -7.923) centre (0, 0) ccw projected
  arc A139 (9.6359, -7.923) -> (9.6254, -7.721) centre (9.5201, -7.8278) ccw projected
  arc A140 (9.4447, -7.4787) -> (9.6254, -7.721) centre (10.3276, -7.009) ccw projected
  arc A141 (10.0312, -6.6715) -> (9.4447, -7.4787) centre (9.9347, -7.218) ccw projected
  arc A142 (10.3175, -6.7684) -> (10.0312, -6.6715) centre (9.8574, -7.6562) ccw projected
  arc A143 (10.3175, -6.7684) -> (10.5129, -6.7159) centre (10.3865, -6.6352) ccw projected
  arc A144 (10.5129, -6.7159) -> (10.7567, -6.3181) centre (0, 0) ccw projected
  arc A145 (10.7567, -6.3181) -> (10.7147, -6.1202) centre (10.6274, -6.2421) ccw projected
  arc A146 (10.4984, -5.9091) -> (10.7147, -6.1202) centre (11.2969, -5.3071) ccw projected
  arc A147 (10.9514, -5.0201) -> (10.4984, -5.9091) centre (10.9416, -5.575) ccw projected
  arc A148 (11.2493, -5.071) -> (10.9514, -5.0201) centre (10.9337, -6.0199) ccw projected
  arc A149 (11.2493, -5.071) -> (11.4341, -4.9887) centre (11.2966, -4.9287) ccw projected
  arc A150 (11.4341, -4.9887) -> (11.6127, -4.5576) centre (0, 0) ccw projected
  arc A151 (11.6127, -4.5576) -> (11.5402, -4.3687) centre (11.473, -4.5028) ccw projected
  arc A152 (11.2935, -4.194) -> (11.5402, -4.3687) centre (11.988, -3.4746) ccw projected
  arc A153 (11.6018, -3.2451) -> (11.2935, -4.194) centre (11.679, -3.7947) ccw projected
  arc A154 (11.9041, -3.2488) -> (11.6018, -3.2451) centre (11.7408, -4.2354) ccw projected
  arc A155 (11.9041, -3.2488) -> (12.0737, -3.1386) centre (11.9286, -3.1008) ccw projected
  arc A156 (12.0737, -3.1386) -> (12.1827, -2.6849) centre (0, 0) ccw projected
  arc A157 (12.1827, -2.6849) -> (12.0815, -2.5096) centre (12.0362, -2.6526) ccw projected
  arc A158 (11.8106, -2.3757) -> (12.0815, -2.5096) centre (12.384, -1.5564) ccw projected
  arc A159 (11.9666, -1.3902) -> (11.8106, -2.3757) centre (12.1288, -1.921) ccw projected
  arc A160 (12.2657, -1.3466) -> (11.9666, -1.3902) centre (12.2588, -2.3466) ccw projected
  arc A161 (12.2657, -1.3466) -> (12.4161, -1.2112) centre (12.2668, -1.1966) ccw projected
  arc A162 (12.4161, -1.2112) -> (12.4527, -0.746) centre (0, 0) ccw projected
  arc A163 (12.4527, -0.746) -> (12.3254, -0.5887) centre (12.3029, -0.7371) ccw projected
  arc A164 (12.0368, -0.4989) -> (12.3254, -0.5887) centre (12.475, 0.4) ccw projected
  arc A165 (12.0368, 0.4989) -> (12.0368, -0.4989) centre (12.28, 0) ccw projected
  arc A166 (12.3254, 0.5887) -> (12.0368, 0.4989) centre (12.475, -0.4) ccw projected
  arc A167 (12.3254, 0.5887) -> (12.4527, 0.746) centre (12.3029, 0.7371) ccw projected
  arc A168 (12.4527, 0.746) -> (12.4161, 1.2112) centre (0, 0) ccw projected
  arc A169 (12.4161, 1.2112) -> (12.2657, 1.3466) centre (12.2668, 1.1966) ccw projected
  arc A170 (11.9666, 1.3902) -> (12.2657, 1.3466) centre (12.2588, 2.3466) ccw projected
  arc A171 (11.8106, 2.3757) -> (11.9666, 1.3902) centre (12.1288, 1.921) ccw projected
  arc A172 (12.0815, 2.5096) -> (11.8106, 2.3757) centre (12.384, 1.5564) ccw projected
  arc A173 (12.0815, 2.5096) -> (12.1827, 2.6849) centre (12.0362, 2.6526) ccw projected
  arc A174 (12.1827, 2.6849) -> (12.0737, 3.1386) centre (0, 0) ccw projected
  arc A175 (12.0737, 3.1386) -> (11.9041, 3.2488) centre (11.9286, 3.1008) ccw projected
  arc A176 (11.6018, 3.2451) -> (11.9041, 3.2488) centre (11.7408, 4.2354) ccw projected
  arc A177 (11.2935, 4.194) -> (11.6018, 3.2451) centre (11.679, 3.7947) ccw projected
  arc A178 (11.5402, 4.3687) -> (11.2935, 4.194) centre (11.988, 3.4746) ccw projected
  arc A179 (11.5402, 4.3687) -> (11.6127, 4.5576) centre (11.473, 4.5028) ccw projected
  arc A180 (11.6127, 4.5576) -> (11.4341, 4.9887) centre (0, 0) ccw projected
  arc A181 (11.4341, 4.9887) -> (11.2493, 5.071) centre (11.2966, 4.9287) ccw projected
  arc A182 (10.9514, 5.0201) -> (11.2493, 5.071) centre (10.9337, 6.0199) ccw projected
  arc A183 (10.4984, 5.9091) -> (10.9514, 5.0201) centre (10.9416, 5.575) ccw projected
  arc A184 (10.7147, 6.1202) -> (10.4984, 5.9091) centre (11.2969, 5.3071) ccw projected
  arc A185 (10.7147, 6.1202) -> (10.7567, 6.3181) centre (10.6274, 6.2421) ccw projected
  arc A186 (10.7567, 6.3181) -> (10.5129, 6.7159) centre (0, 0) ccw projected
  arc A187 (10.5129, 6.7159) -> (10.3175, 6.7684) centre (10.3865, 6.6352) ccw projected
  arc A188 (10.0312, 6.6715) -> (10.3175, 6.7684) centre (9.8574, 7.6562) ccw projected
  arc A189 (9.4447, 7.4787) -> (10.0312, 6.6715) centre (9.9347, 7.218) ccw projected
  arc A190 (9.6254, 7.721) -> (9.4447, 7.4787) centre (10.3276, 7.009) ccw projected
  arc A191 (9.6254, 7.721) -> (9.6359, 7.923) centre (9.5201, 7.8278) ccw projected
  arc A192 (9.6359, 7.923) -> (9.3329, 8.2778) centre (0, 0) ccw projected
  arc A193 (9.3329, 8.2778) -> (9.1317, 8.2991) centre (9.2207, 8.1783) ccw projected
  arc A194 (8.8641, 8.1585) -> (9.1317, 8.2991) centre (8.5383, 9.104) ccw projected
  arc A195 (8.1585, 8.8641) -> (8.8641, 8.1585) centre (8.6833, 8.6833) ccw projected
  arc A196 (8.2991, 9.1317) -> (8.1585, 8.8641) centre (9.104, 8.5383) ccw projected
  arc A197 (8.2991, 9.1317) -> (8.2778, 9.3329) centre (8.1783, 9.2207) ccw projected
  arc A198 (8.2778, 9.3329) -> (7.923, 9.6359) centre (0, 0) ccw projected
  arc A199 (7.923, 9.6359) -> (7.721, 9.6254) centre (7.8278, 9.5201) ccw projected
  arc A200 (7.4787, 9.4447) -> (7.721, 9.6254) centre (7.009, 10.3276) ccw projected
  arc A201 (6.6715, 10.0312) -> (7.4787, 9.4447) centre (7.218, 9.9347) ccw projected
  arc A202 (6.7684, 10.3175) -> (6.6715, 10.0312) centre (7.6562, 9.8574) ccw projected
  arc A203 (6.7684, 10.3175) -> (6.7159, 10.5129) centre (6.6352, 10.3865) ccw projected
  arc A204 (6.7159, 10.5129) -> (6.3181, 10.7567) centre (0, 0) ccw projected
  arc A205 (6.3181, 10.7567) -> (6.1202, 10.7147) centre (6.2421, 10.6274) ccw projected
  arc A206 (5.9091, 10.4984) -> (6.1202, 10.7147) centre (5.3071, 11.2969) ccw projected
  arc A207 (5.0201, 10.9514) -> (5.9091, 10.4984) centre (5.575, 10.9416) ccw projected
  arc A208 (5.071, 11.2493) -> (5.0201, 10.9514) centre (6.0199, 10.9337) ccw projected
  arc A209 (5.071, 11.2493) -> (4.9887, 11.4341) centre (4.9287, 11.2966) ccw projected
  arc A210 (4.9887, 11.4341) -> (4.5576, 11.6127) centre (0, 0) ccw projected
  arc A211 (4.5576, 11.6127) -> (4.3687, 11.5402) centre (4.5028, 11.473) ccw projected
  arc A212 (4.194, 11.2935) -> (4.3687, 11.5402) centre (3.4746, 11.988) ccw projected
  arc A213 (3.2451, 11.6018) -> (4.194, 11.2935) centre (3.7947, 11.679) ccw projected
  arc A214 (3.2488, 11.9041) -> (3.2451, 11.6018) centre (4.2354, 11.7408) ccw projected
  arc A215 (3.2488, 11.9041) -> (3.1386, 12.0737) centre (3.1008, 11.9286) ccw projected
  arc A216 (3.1386, 12.0737) -> (2.6849, 12.1827) centre (0, 0) ccw projected
  arc A217 (2.6849, 12.1827) -> (2.5096, 12.0815) centre (2.6526, 12.0362) ccw projected
  arc A218 (2.3757, 11.8106) -> (2.5096, 12.0815) centre (1.5564, 12.384) ccw projected
  arc A219 (1.3902, 11.9666) -> (2.3757, 11.8106) centre (1.921, 12.1288) ccw projected
  arc A220 (1.3466, 12.2657) -> (1.3902, 11.9666) centre (2.3466, 12.2588) ccw projected
  arc A221 (1.3466, 12.2657) -> (1.2112, 12.4161) centre (1.1966, 12.2668) ccw projected
  arc A222 (1.2112, 12.4161) -> (0.746, 12.4527) centre (0, 0) ccw projected
  arc A223 (0.746, 12.4527) -> (0.5887, 12.3254) centre (0.7371, 12.3029) ccw projected
  arc A224 (0.4989, 12.0368) -> (0.5887, 12.3254) centre (-0.4, 12.475) ccw projected
  arc A225 (-0.4989, 12.0368) -> (0.4989, 12.0368) centre (0, 12.28) ccw projected
  arc A226 (-0.5887, 12.3254) -> (-0.4989, 12.0368) centre (0.4, 12.475) ccw projected
  arc A227 (-0.5887, 12.3254) -> (-0.746, 12.4527) centre (-0.7371, 12.3029) ccw projected
  arc A228 (-0.746, 12.4527) -> (-1.2112, 12.4161) centre (0, 0) ccw projected
  arc A229 (-1.2112, 12.4161) -> (-1.3466, 12.2657) centre (-1.1966, 12.2668) ccw projected
  arc A230 (-1.3902, 11.9666) -> (-1.3466, 12.2657) centre (-2.3466, 12.2588) ccw projected
  arc A231 (-2.3757, 11.8106) -> (-1.3902, 11.9666) centre (-1.921, 12.1288) ccw projected
  arc A232 (-2.5096, 12.0815) -> (-2.3757, 11.8106) centre (-1.5564, 12.384) ccw projected
  arc A233 (-2.5096, 12.0815) -> (-2.6849, 12.1827) centre (-2.6526, 12.0362) ccw projected
  arc A234 (-2.6849, 12.1827) -> (-3.1386, 12.0737) centre (0, 0) ccw projected
  arc A235 (-3.1386, 12.0737) -> (-3.2488, 11.9041) centre (-3.1008, 11.9286) ccw projected
  arc A236 (-3.2451, 11.6018) -> (-3.2488, 11.9041) centre (-4.2354, 11.7408) ccw projected
  arc A237 (-4.194, 11.2935) -> (-3.2451, 11.6018) centre (-3.7947, 11.679) ccw projected
  arc A238 (-4.3687, 11.5402) -> (-4.194, 11.2935) centre (-3.4746, 11.988) ccw projected
  arc A239 (-4.3687, 11.5402) -> (-4.5576, 11.6127) centre (-4.5028, 11.473) ccw projected
  point P0 (0, 0)
